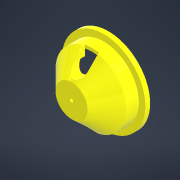
# Autodesk Inventor part: 016
Saved by Autodesk Inventor 2022 (Build 260153000, 153)
## iProperties
Created: 2021-11-15
Part Number: 016
Material: Stainless Steel, Austenitic
Document SubType Name: Modeling
Designer: vinicius.miguel
Density: 8 g/cm^3
Appearance: Smooth - Yellow
Mass: 11.4343 g
Surface Area: 20.6833 cm^2
Volume: 1.42929 cm^3
Author: vinicius.miguel
Autodesk Inventor part; units mm, degrees
ref_plane "YZ Plane" through (0, 0, 0) normal (1, 0, 0) x (0, 1, 0)
ref_plane "XZ Plane" through (0, 0, 0) normal (0, 1, 0) x (-1, 0, 0)
sketch "Sketch1" plane through (0, 0, 0) normal (0, 1, 0) x (-1, 0, 0)
  line L0 (1.366, -1) -> (4.5858, -1)
  line L1 (5, 0) -> (0.5, 0)
  line L2 (4.5858, -1) -> (10, -6.4142)
  line L3 (5, 0) -> (11, -6)
  line L4 (11, -6) -> (11, -10)
  line L5 (11, -10) -> (13, -10)
  line L6 (13, -10) -> (13, -11.5)
  line L7 (13, -11.5) -> (10, -11.5)
  line L8 (10, -11.5) -> (10, -6.4142)
  line L9 (0, 0) -> (0, -4.2235)
  line L10 (10, -6.4142) -> (1.366, -6.4142)
  line L11 (1.366, -6.4142) -> (1.366, -1)
  line L12 (0.5, 0) -> (0.5, -0.5)
  line L13 (0.5, -0.5) -> (1.366, -1)
  dimension "d3" = 26
  dimension "d5" = 20
  dimension "d6" = 1
  dimension "d7" = 135
  dimension "d8" = 1
  dimension "d9" = 10
  dimension "d10" = 11.5
  dimension "d11" = 1.5
  dimension "d32" = 1
  dimension "d33" = 1
  dimension "d34" = 0.5
  dimension "d35" = 30
  constraints: 28 end point, 6 perpendicular, 3 vertical, 2 parallel, 1 horizontal, 1 horizontal alignment
  measures "d3" diameter of L6 L9
  measures "d5" diameter of L8 L9
  measures "d6" distance between parallel lines of L4 L8
  measures "d7" angle of L2 L0
  measures "d8" distance between parallel lines of L3 L2
  measures "d9" diameter of L1.start L9
  measures "d10" distance from line of L7 L9.start
  measures "d11" distance between parallel lines of L7 L5
  measures "d32" diameter of L12 L9
  measures "d33" distance between parallel lines of L1 L0
  measures "d34" distance of L1.end L12.end
  measures "d35" angle of L13 L0
revolve "Revolution1" add sketch "Sketch1" angle 360 about axis through (0, 0, 0) along (0, 0, -1)
sketch "Sketch4" plane through (0, 0, -6.4142) normal (0, 0, -1) x (-1, 0, 0)
  circle A0 centre (0, 0) radius 1.366 projected
  constraints: 1 coincident
hole "Hole2" at (0, 0, -6.4142) direction (0, 0, 1) diameter 16 depth 1.4 tip angle 118
ref_plane "Work Plane2" through (0, 0, -6.4142) normal (0, 0, -1) x (-1, 0, 0)
sketch "Sketch5" plane through (0, 0, -6.4142) normal (0, 0, -1) x (-1, 0, 0)
  circle A0 centre (0, 0) radius 10 projected
  line L0 (0, -13.75) -> (0, -7.75) construction
  line L1 (2.25, -13.75) -> (2.25, -7.75)
  line L2 (-2.25, -7.75) -> (-2.25, -13.75)
  arc A1 (-2.25, -13.75) -> (2.25, -13.75) centre (0, -13.75) ccw
  arc A2 (2.25, -7.75) -> (-2.25, -7.75) centre (0, -7.75) ccw
  point P0 (0, -10.75)
  dimension "d37" = 4.5
  dimension "d38" = 6
  constraints: 8 end point, 5 tangent, 4 point on circle, 2 centre point, 1 midpoint, 1 parallel, 1 vertical, 1 vertical alignment
  measures "d37" diameter of A2
  measures "d38" distance of L2.start L2.end
extrude "Extrusion1" cut sketch "Sketch5" against normal blind 10 contours L2 A2 L1 A0 | A0 L1 A1 L2 picked at (-0.2519, -8.4905)
pattern_circular "Circular Pattern2" count 2 over 360 about axis through (0, 0, -8) along (0, 0, -1) of "Extrusion1"
body "Solid1"
